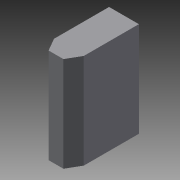
# Autodesk Inventor part: interior case
Saved by Autodesk Inventor 2013 (Build 170138000, 138)
## iProperties
Created: 2014-06-26
Part Number: interior case
Material: Genérico
Document SubType Name: Chapa
Designer: Administrador
Density: 1 g/cm^3
Sheet Metal Rule: Por defecto_mm
Author: Administrador
Autodesk Inventor part; units mm, degrees
ref_plane "YZ Plane" through (0, 0, 0) normal (1, 0, 0) x (0, 1, 0)
ref_plane "XZ Plane" through (0, 0, 0) normal (0, 1, 0) x (-1, 0, 0)
ref_plane "XY Plane" through (0, 0, 0) normal (0, 0, 1) x (1, 0, 0)
sketch "Boceto1" plane through (0, 0, 0) normal (0, 0, 1) x (1, 0, 0)
  line L0 (10.3987, 16.5828) -> (-9.2013, 16.5828)
  line L1 (-9.2013, -19.6772) -> (-9.2013, 16.5828)
  line L2 (-4.3013, -28.1643) -> (-9.2013, -19.6772)
  line L3 (5.4987, -28.1643) -> (-4.3013, -28.1643)
  line L4 (10.3987, -19.6772) -> (5.4987, -28.1643)
  line L5 (10.3987, 16.5828) -> (10.3987, -19.6772)
  constraints: 12 end point
extrude "Extrusión1" add sketch "Boceto1" along normal blind 62.5
shell "Vaciado1" thickness 1 removed faces 1 at (-2.668, -7.5906, 0)
equation "\"Radio_pliegue\" = Grosor"
equation "\"Anchura_desahogo_plegado\" = Grosor"
equation "\"Profundidad_desahogo_plegado\" = 0.5 * Grosor"
equation "\"Tamaño_destalonado\" = 4 * Grosor"
equation "\"Remanente_mínimo\" = 2 * Grosor"
equation "\"Radiodetransición\" = Radio_pliegue"
equation "\"Tamaño_de_radio_de_Jacobi\" = Radio_pliegue"
equation "\"TamañoSeparación\" = Grosor"
equation "\"Grosor\" = 0.5"
